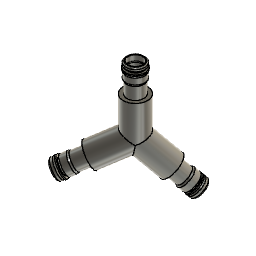
Derivação em Y v2 (Autodesk Fusion 360 design; units mm, degrees)
Autodesk Fusion 360 part; units mm, degrees
sketch "Sketch1" plane through (0, 0, 0) normal (0, 0, 1) x (1, 0, 0)
  circle A0 centre (0, 0) radius 10
  dimension "d1" = 20
  constraint coincident A0.centre origin
  measures "d1" diameter of A0
extrude "Extrude1" add sketch "Sketch1" along normal blind 30
sketch "Sketch2" plane through (0, 0, 0) normal (0, 0, -1) x (1, 0, 0)
  circle A0 centre (0, 0) radius 10
  circle A1 through (7.0711, 7.0711, 0) (-7.8657, 0.7946, 6.1237) (0.7946, -7.8657, -6.1237) construction
  circle A2 through (-7.0711, -7.0711, 0) (-0.7946, 7.8657, 6.1237) (7.8657, -0.7946, -6.1237)
extrude "Extrude2" add sketch "Sketch2" along normal blind 30 contours A2 in plane through (0, 0, 0) normal (0.5, 0.5, -0.707107)
sketch "Sketch3" plane through (0, 0, 0) normal (0, 0, -1) x (1, 0, 0)
sketch "Sketch4" plane through (0, 0, 0) normal (0, 0, 1) x (1, 0, 0)
  circle A0 through (-3.0868, -3.4503, 8.8638) (7.6906, -4.3706, -4.664) (-4.6038, 7.8209, -4.1998)
  dimension "d6" = 20
extrude "Extrude3" add sketch "Sketch4" against normal blind 30 contours A0 in plane through (0, 0, 0) normal (0.633151, 0.620891, 0.462185)
sketch "Sketch5" plane through (0, 0, 30) normal (0, 0, 1) x (-1, 0, 0)
  circle A0 centre (0, 0) radius 10
  circle A1 centre (0, 0) radius 7
  dimension "d9" = 14
  constraint coincident A0.centre A1.centre
  measures "d9" diameter of A1
extrude "Extrude4" add sketch "Sketch5" along normal blind 10 contours A1
sketch "Sketch6" plane through (0, 0, 40) normal (0, 0, 1) x (-1, 0, 0)
  circle A0 centre (0, 0) radius 7
extrude "Extrude5" add sketch "Sketch6" along normal blind 1.5 draft 25
extrude "Extrude6" add 1 faces at (-1.895, -0.0503, 41.5) along direction (0, 0, 1) blind 3.5
extrude "Extrude7" add 1 faces at (-1.895, -0.0503, 45) along direction (0, 0, 1) blind 1.5
extrude "Extrude8" add 1 faces at (-1.895, -0.0503, 46.5) along direction (0, 0, 1) blind 1.5 draft -45
sketch "Sketch7" plane through (0, 0, 48) normal (0, 0, 1) x (-1, 0, 0)
  circle A0 centre (0, 0) radius 6.1995
  circle A1 centre (0, 0) radius 8.0695
  constraint coincident A0.centre A1.centre
extrude "Extrude9" add sketch "Sketch7" along normal blind 1 contours A0 | A1
sketch "Sketch8" plane through (0, 0, 49) normal (0, 0, 1) x (-1, 0, 0)
  circle A0 centre (0, 0) radius 8.0695
  circle A1 centre (0, 0) radius 6.1995
  dimension "d22" = 12.399
  constraint coincident A0.centre A1.centre
  measures "d22" diameter of A1
extrude "Extrude10" add sketch "Sketch8" along normal blind 1.5 draft 45 contours A1
extrude "Extrude11" add 1 faces at (1.2276, -4.6303, 50.5) along direction (0, 0, 1) blind 3
fillet "Fillet1" radius 1 1 edges at (7.1785, 2.7843, 53.5)
fillet "Fillet1" radius 1 1 edges at (7.1785, -2.7843, 50.5)
hole "Hole1" at (0, 0, 53.5) direction (0, 0, -1) diameter 12 depth 54 tip angle 180
sketch "Sketch9" plane through (15, 15, -21.2132) normal (0.5, 0.5, -0.707107) x (-0.707107, 0.707107, 0)
  circle A0 centre (0, 0) radius 10
  circle A1 centre (0, 0) radius 7
  dimension "d34" = 14
  constraint coincident A0.centre A1.centre
  measures "d34" diameter of A1
extrude "Extrude12" add sketch "Sketch9" along normal blind 10 contours A1
extrude "Extrude13" add 1 faces at (22.8577, 19.0354, -26.9456) along direction (0.5, 0.5, -0.707107) blind 1.5 draft 25
extrude "Extrude14" add 1 faces at (18.5277, 21.5266, -30.3672) along direction (0.5, 0.5, -0.707107) blind 5
extrude "Extrude15" add 1 faces at (21.0277, 24.0266, -33.9028) along direction (0.5, 0.5, -0.707107) blind 1.5 draft -45
sketch "Sketch10" plane through (24, 24, -33.9411) normal (0.5, 0.5, -0.707107) x (-0.707107, 0.707107, 0)
  circle A0 centre (0, 0) radius 6.1995
  circle A1 centre (0, 0) radius 7.1995
  circle A2 centre (0, 0) radius 7.6995
  dimension "d43" = 14.399
  dimension "d44" = 15.399
  constraint coincident A0.centre A1.centre
  measures "d43" diameter of A1
  measures "d44" diameter of A2
extrude "Extrude16" add sketch "Sketch10" along normal blind 1 contours A0 | A1 | A2
sketch "Sketch11" plane through (24.5, 24.5, -34.6482) normal (0.5, 0.5, -0.707107) x (-0.707107, 0.707107, 0)
  circle A0 centre (0, 0) radius 7.6995
  circle A1 centre (0, 0) radius 6.1995
  dimension "d47" = 12.399
  constraint coincident A0.centre A1.centre
  measures "d47" diameter of A1
extrude "Extrude17" add sketch "Sketch11" along normal blind 1.5 draft 45 contours A1
extrude "Extrude18" add 1 faces at (25.0423, 27.1072, -34.5425) along direction (0.5, 0.5, -0.707107) blind 3
fillet "Fillet2" radius 1 1 edges at (30.4338, 20.2819, -39.799)
sketch "Sketch12" plane through (-18.9945, -18.6267, -13.8655) normal (-0.633151, -0.620891, -0.462185) x (0.700161, -0.713985, 0)
  circle A0 centre (0, 0) radius 10
  circle A1 centre (0, 0) radius 7
  dimension "d54" = 14
  constraint coincident A0.centre A1.centre
  measures "d54" diameter of A1
extrude "Extrude19" add sketch "Sketch12" along normal blind 10 contours A1
extrude "Extrude20" add 1 faces at (-27.1005, -25.1214, -15.6726) along direction (-0.633151, -0.620891, -0.462185) blind 1.5 draft 20
extrude "Extrude21" add 1 faces at (-25.3322, -24.5784, -22.0699) along direction (-0.633151, -0.620891, -0.462185) blind 5
extrude "Extrude22" add 1 faces at (-28.498, -27.6829, -24.3808) along direction (-0.633151, -0.620891, -0.462185) blind 1.5 draft -45
sketch "Sketch13" plane through (-30.3912, -29.8028, -22.1849) normal (-0.633151, -0.620891, -0.462185) x (0.700161, -0.713985, 0)
  circle A0 centre (0, 0) radius 6.046
  circle A1 centre (0, 0) radius 8.0695
  dimension "d63" = 16.139
  constraint coincident A0.centre A1.centre
  measures "d63" diameter of A1
extrude "Extrude23" add sketch "Sketch13" along normal blind 1 contours A0 | A1
sketch "Sketch14" plane through (-31.0244, -30.4237, -22.6471) normal (-0.633151, -0.620891, -0.462185) x (0.700161, -0.713985, 0)
  circle A0 centre (0, 0) radius 8.0695
  circle A1 centre (0, 0) radius 6.1995
  dimension "d66" = 12.399
  constraint coincident A0.centre A1.centre
  measures "d66" diameter of A1
extrude "Extrude24" add sketch "Sketch14" along normal blind 1.5 draft 45 contours A1
extrude "Extrude25" add 1 faces at (-32.6355, -29.6929, -24.667) along direction (-0.633151, -0.620891, -0.462185) blind 3
fillet "Fillet3" radius 1 1 edges at (-37.9808, -27.1914, -27.1959)
hole "Hole2" at (-33.8736, -33.2177, -24.7269) direction (0.633151, 0.620891, 0.462185) diameter 12 depth 54 tip angle 180
hole "Hole3" at (26.75, 26.75, -37.8302) direction (-0.5, -0.5, 0.707107) diameter 12 depth 54 tip angle 180
